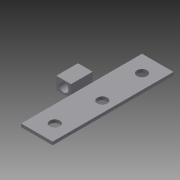
# Autodesk Inventor part: door hinge for conveyor part 2
Saved by Autodesk Inventor 2015 (Build 190159000, 159)
## iProperties
Created: 2015-02-03
Part Number: door hinge for conveyor part 2
Material: Generic
Document SubType Name: Modeling
Designer: szymsea16
Density: 1 g/cm^3
Appearance: Default
Author: szymsea16
Autodesk Inventor part; units mm, degrees
ref_plane "YZ Plane" through (0, 0, 0) normal (1, 0, 0) x (0, 1, 0)
ref_plane "XZ Plane" through (0, 0, 0) normal (0, 1, 0) x (-1, 0, 0)
ref_plane "XY Plane" through (0, 0, 0) normal (0, 0, 1) x (1, 0, 0)
sketch "Sketch1" plane through (0, 0, 0) normal (0, 1, 0) x (-1, 0, 0)
  line L0 (0, 0) -> (0, -63.881)
  line L1 (0, -63.881) -> (16.891, -63.881)
  line L2 (16.891, -63.881) -> (16.891, 0)
  line L3 (16.891, 0) -> (0, 0)
  line L4 (16.891, 0) -> (24.638, 0)
  line L5 (24.638, 0) -> (24.638, -11.43)
  line L6 (24.638, -11.43) -> (16.891, -11.43)
  line L7 (16.891, -63.881) -> (24.638, -63.881)
  line L8 (24.638, -63.881) -> (24.638, -52.451)
  line L9 (24.638, -52.451) -> (16.891, -52.451)
  dimension "d0" = 63.881
  dimension "d1" = 16.891
  dimension "d2" = 7.747
  dimension "d3" = 11.43
  dimension "d4" = 7.747
  dimension "d5" = 11.43
  constraints: 20 end point, 6 perpendicular, 5 point on line, 1 vertical
  measures "d0" distance of L0.start L0.end
  measures "d1" distance of L0.end L1.end
  measures "d2" distance of L2.end L4.end
  measures "d3" distance of L4.end L5.end
  measures "d4" distance of L1.end L7.end
  measures "d5" distance of L7.end L8.end
extrude "Extrusion1" add sketch "Sketch1" along normal blind 1.651 contours L3 L2 L1 L0
hole "Hole3" at (-5.715, 1.651, -32.131) direction (0, -1, 0) diameter 5.334 end through all
sketch "Sketch2" plane through (0, 1.651, 0) normal (0, 1, 0) x (1, 0, 0)
  line L0 (-16.891, 63.881) -> (-16.891, 31.9405)
  line L1 (-16.891, 63.881) -> (-16.891, 0) projected
  line L2 (-16.891, 31.9405) -> (-16.891, 37.6555)
  line L3 (-16.891, 37.6555) -> (-24.638, 37.6555)
  line L4 (-24.638, 37.6555) -> (-24.638, 26.2255)
  line L5 (-24.638, 26.2255) -> (-16.891, 26.2255)
  line L6 (-16.891, 31.9405) -> (-16.891, 37.6555)
  point P0 (0, 0)
  dimension "d48" = 31.9405
  dimension "d49" = 5.715
  dimension "d50" = 7.747
  dimension "d51" = 11.43
  constraints: 12 end point, 3 perpendicular, 2 point on line, 1 collinear, 1 midpoint
  measures "d48" distance of L0.start L0.end
  measures "d49" distance of L0.end L2.end
  measures "d50" distance of L2.end L3.end
  measures "d51" distance of L3.end L4.end
extrude "Extrusion4" add sketch "Sketch2" along normal blind 6.477
hole "Hole5" at (-20.7645, 4.8895, -26.2255) direction (0, 0, -1) diameter 5.08 end through all
sketch "Sketch3" plane through (0, 1.651, 0) normal (0, 1, 0) x (1, 0, 0)
  line L0 (0, 63.881) -> (-16.891, 63.881)
  line L1 (-16.891, 63.881) -> (-16.891, 0)
  line L2 (-16.891, 0) -> (0, 0)
  line L3 (0, 0) -> (0, 63.881)
  line L4 (0, 63.881) -> (-16.891, 63.881) projected
  constraints: 8 end point, 3 perpendicular, 1 horizontal
extrude "Extrusion5" cut sketch "Sketch3" against normal blind 6.35
sketch "Sketch4" plane through (-16.891, 1.651, -37.6555) normal (1, 0, 0) x (0, 0, -1)
  line L0 (0, 0) -> (-11.43, 0) projected
  line L1 (-5.715, 0) -> (26.0985, 0)
  line L2 (26.0985, 0) -> (26.0985, 1.651)
  line L3 (26.0985, 0) -> (26.0985, 1.651)
  line L4 (26.0985, 1.651) -> (-37.7825, 1.651)
  line L5 (-37.7825, 1.651) -> (-37.7825, 0)
  line L6 (-37.7825, 0) -> (-11.43, 0)
  point P0 (-37.6555, -1.651)
  dimension "d65" = 31.8135
  dimension "d66" = 1.651
  dimension "d67" = 1.651
  dimension "d68" = 63.881
  constraints: 12 end point, 3 perpendicular, 1 collinear, 1 horizontal, 1 midpoint, 1 vertical
  measures "d65" distance of L1.start L1.end
  measures "d66" distance of L1.end L2.end
  measures "d67" distance of L1.end L2.end
  measures "d68" distance of L2.end L4.end
extrude "Extrusion6" add sketch "Sketch4" along normal blind 16.637
hole "Hole6" at (-8.001, 3.302, -8.763) direction (0, -1, 0) diameter 5.334 end through all
hole "Hole7" at (-8.001, 3.302, -54.864) direction (0, -1, 0) diameter 5.334 end through all
hole "Hole8" at (-5.969, 3.302, -31.8135) direction (0, -1, 0) diameter 5.334 end through all
body "Solid1"
